LGR Coupler Bracket (Defensemen) (Autodesk Fusion 360 design; units mm, degrees)
Autodesk Fusion 360 part; units mm, degrees
sketch "Sketch1" plane through (0, 0, 0) normal (0, 0, 1) x (1, 0, 0)
  line L0 (-26.575, 21) -> (26.575, 21)
  line L1 (26.575, 21) -> (26.575, -21)
  line L2 (26.575, -21) -> (-26.575, -21)
  line L3 (-26.575, -21) -> (-26.575, 21)
  dimension "d2" = 53.15
  dimension "d3" = 42
  dimension "d4" = 21
  dimension "d5" = 26.575
  constraint horizontal L0
  constraint vertical L1
  constraint horizontal L2
  constraint vertical L3
  measures "d2" distance of L1 L3
  measures "d3" distance of L0 L2
  measures "d4" distance of origin L0
  measures "d5" distance of origin L1
extrude "Extrude1" add sketch "Sketch1" along normal blind 6 makes body 1
sketch "Sketch2" plane through (0, 0, 6) normal (0, 0, 1) x (-1, 0, 0)
  line L0 (26.575, 21) -> (-26.575, 21)
  line L1 (-26.575, 21) -> (-26.575, -21)
  line L2 (-26.575, -21) -> (26.575, -21)
  line L3 (26.575, -21) -> (26.575, 21)
  point P0 (20.01, -13)
  point P1 (-19.99, -13)
  point P2 (20.01, -1)
  point P3 (-19.99, -1)
  dimension "d8" = 40
  dimension "d9" = 12
  dimension "d10" = 6.565
  dimension "d11" = 22
  constraint horizontal P0 P1
  constraint vertical P1 P3
  constraint horizontal P2 P3
  constraint vertical P0 P2
  measures "d8" distance of P0 P1
  measures "d9" distance of P1 P3
  measures "d10" distance of L3 P0
  measures "d11" distance of L0 P2
hole "Hole1" at (-20.01, 13, 6) at (-20.01, 1, 6) at (19.99, 13, 6) at (19.99, 1, 6) direction (0, 0, -1) diameter 5.5 depth 10 tip angle 180 counterbore diameter 10 counterbore depth 5 bodies 1
sketch "Sketch3" plane through (0, 0, 6) normal (0, 0, 1) x (-1, 0, 0)
  circle A0 centre (-19.99, -13) radius 5
  circle A1 centre (20.01, -13) radius 5
  circle A2 centre (20.01, -1) radius 5
  circle A3 centre (-19.99, -1) radius 5
  line L0 (26.575, 21) -> (-26.575, 21)
  line L1 (-26.575, 21) -> (-26.575, -21)
  line L2 (-26.575, -21) -> (26.575, -21)
  line L3 (26.575, -21) -> (26.575, 21)
  circle A4 centre (0.01, -7) radius 12.7
  dimension "d17" = 25.4
  dimension "d18" = 20
  dimension "d19" = 6
  measures "d17" diameter of A4
  measures "d18" horizontal distance of A2.centre A4.centre
  measures "d19" vertical distance of A1.centre A4.centre
extrude "Extrude2" cut sketch "Sketch3" against normal blind 6 contours A4 bodies 1
sketch "Sketch4" plane through (0, 0, 0) normal (0, 0, -1) x (1, 0, 0)
  circle A0 centre (-0.01, -7) radius 12.7
  circle A1 centre (19.99, -13) radius 2.75
  circle A2 centre (-20.01, -13) radius 2.75
  circle A3 centre (-20.01, -1) radius 2.75
  circle A4 centre (19.99, -1) radius 2.75
  line L0 (26.575, 21) -> (-26.575, 21)
  line L1 (-26.575, 21) -> (-26.575, -21)
  line L2 (-26.575, -21) -> (26.575, -21)
  line L3 (26.575, -21) -> (26.575, 21)
  circle A5 centre (-0.01, -7) radius 12.7
  circle A6 centre (-0.01, -7) radius 15.875
  dimension "d22" = 25.4
  dimension "d23" = 31.75
  constraint concentric A0 A5
  constraint concentric A5 A6
  measures "d22" diameter of A5
  measures "d23" diameter of A6
extrude "Extrude3" add sketch "Sketch4" along normal blind 1.25 contours L2 A6 | L2 A6 bodies 1
ref_plane "WorkPlane1" through (0, 0, 49) normal (0, 0, 1) x (1, 0, 0)
sketch "Sketch5" plane through (0, 0, 49) normal (0, 0, 1) x (1, 0, 0)
  line L0 (-28.5, 36) -> (28.5, 36)
  line L1 (28.5, 36) -> (28.5, -21)
  line L2 (28.5, -21) -> (-28.5, -21)
  line L3 (-28.5, -21) -> (-28.5, 36)
  point P0 (-26.575, -21)
  dimension "d27" = 57
  dimension "d28" = 57
  dimension "d29" = 28.5
  constraint horizontal L0
  constraint vertical L1
  constraint horizontal L2
  constraint vertical L3
  constraint horizontal L2.end P0
  measures "d27" distance of L0 L2
  measures "d28" distance of L1 L3
  measures "d29" distance of origin L3
extrude "Extrude4" add sketch "Sketch5" against normal blind 6 separate body makes body 2
sketch "Sketch6" plane through (0, 0, 49) normal (0, 0, 1) x (-1, 0, 0)
  line L0 (28.5, 21) -> (-28.5, 21)
  line L1 (-28.5, 21) -> (-28.5, -36)
  line L2 (-28.5, -36) -> (28.5, -36)
  line L3 (28.5, -36) -> (28.5, 21)
  circle A0 centre (0, -7.5) radius 19.1
  dimension "d32" = 38.2
  dimension "d33" = 28.5
  dimension "d34" = 28.5
  measures "d32" diameter of A0
  measures "d33" distance of L0 A0.centre
  measures "d34" distance of L1 A0.centre
extrude "Extrude5" cut sketch "Sketch6" against normal blind 6 contours A0 bodies 2
sketch "Sketch7" plane through (0, 0, 43) normal (0, 0, -1) x (1, 0, 0)
  circle A0 centre (0, -7.5) radius 19.1
  line L0 (28.5, 21) -> (-28.5, 21)
  line L1 (-28.5, 21) -> (-28.5, -36)
  line L2 (-28.5, -36) -> (28.5, -36)
  line L3 (28.5, -36) -> (28.5, 21)
  line L4 (28.5, -36) -> (18.64, -36)
  line L5 (18.64, -36) -> (18.64, -26.14)
  line L6 (18.64, -26.14) -> (28.5, -26.14)
  line L7 (28.5, -26.14) -> (28.5, -36)
  line L8 (-28.5, -36) -> (-18.64, -36)
  line L9 (-18.64, -36) -> (-18.64, -26.14)
  line L10 (-18.64, -26.14) -> (-28.5, -26.14)
  line L11 (-28.5, -26.14) -> (-28.5, -36)
  line L12 (-28.5, 21) -> (-18.64, 21)
  line L13 (-18.64, 21) -> (-18.64, 11.14)
  line L14 (-18.64, 11.14) -> (-28.5, 11.14)
  line L15 (-28.5, 11.14) -> (-28.5, 21)
  line L16 (28.5, 21) -> (18.64, 21)
  line L17 (18.64, 21) -> (18.64, 11.14)
  line L18 (18.64, 11.14) -> (28.5, 11.14)
  line L19 (28.5, 11.14) -> (28.5, 21)
  dimension "d41" = 9.86
  dimension "d42" = 9.86
  dimension "d43" = 9.86
  dimension "d44" = 9.86
  constraint horizontal L4
  constraint vertical L5
  constraint horizontal L6
  constraint vertical L7
  constraint coincident L2.end L3.start
  constraint horizontal L8
  constraint vertical L9
  constraint horizontal L10
  constraint vertical L11
  constraint coincident L1.end L2.start
  constraint horizontal L12
  constraint vertical L13
  constraint horizontal L14
  constraint vertical L15
  constraint coincident L0.end L1.start
  constraint horizontal L16
  constraint vertical L17
  constraint horizontal L18
  constraint vertical L19
  constraint coincident L0.start L3.end
  constraint horizontal L5.end L9.end
  constraint vertical L5.end L17.end
  constraint horizontal L13.end L17.end
  constraint vertical L9.end L13.end
  measures "d41" distance of L5 L7
  measures "d42" distance of L4 L6
  measures "d43" distance of L16 L18
  measures "d44" distance of L13 L15
sketch "Sketch9" plane through (0, 0, 6) normal (0, 0, 1) x (-1, 0, 0)
  circle A0 centre (0.01, -7) radius 12.7
  circle A1 centre (-19.99, -13) radius 5
  circle A2 centre (20.01, -13) radius 5
  circle A3 centre (20.01, -1) radius 5
  circle A4 centre (-19.99, -1) radius 5
  line L0 (26.575, 21) -> (-26.575, 21)
  line L1 (-26.575, 21) -> (-26.575, -21)
  line L2 (-26.575, -21) -> (26.575, -21)
  line L3 (26.575, -21) -> (26.575, 21)
  line L4 (26.575, -21) -> (21.575, -21)
  line L5 (21.575, -21) -> (21.575, -16)
  line L6 (21.575, -16) -> (26.575, -16)
  line L7 (26.575, -16) -> (26.575, -21)
  line L8 (26.575, 21) -> (21.575, 21)
  line L9 (21.575, 21) -> (21.575, 16)
  line L10 (21.575, 16) -> (26.575, 16)
  line L11 (26.575, 16) -> (26.575, 21)
  line L12 (-26.575, -21) -> (-21.575, -21)
  line L13 (-21.575, -21) -> (-21.575, -16)
  line L14 (-21.575, -16) -> (-26.575, -16)
  line L15 (-26.575, -16) -> (-26.575, -21)
  line L16 (-26.575, 21) -> (-21.575, 21)
  line L17 (-21.575, 21) -> (-21.575, 16)
  line L18 (-21.575, 16) -> (-26.575, 16)
  line L19 (-26.575, 16) -> (-26.575, 21)
  dimension "d45" = 5
  dimension "d46" = 5
  dimension "d47" = 5
  dimension "d48" = 5
  constraint horizontal L4
  constraint vertical L5
  constraint horizontal L6
  constraint vertical L7
  constraint coincident L2.end L3.start
  constraint horizontal L8
  constraint vertical L9
  constraint horizontal L10
  constraint vertical L11
  constraint coincident L0.start L3.end
  constraint horizontal L12
  constraint vertical L13
  constraint horizontal L14
  constraint vertical L15
  constraint coincident L1.end L2.start
  constraint horizontal L16
  constraint vertical L17
  constraint horizontal L18
  constraint vertical L19
  constraint coincident L0.end L1.start
  constraint horizontal L5.end L13.end
  constraint vertical L5.end L9.end
  constraint horizontal L9.end L17.end
  constraint vertical L13.end L17.end
  measures "d45" distance of L5 L7
  measures "d46" distance of L4 L6
  measures "d47" distance of L8 L10
  measures "d48" distance of L17 L19
loft "Loft1" add profiles "Sketch7", "Sketch9" section 1 contours L0 L3 L16 L17 L18 L19 section 2 contours L0 L1 L16 L17 L18 L19 bodies 1 2
loft "Loft2" add profiles "Sketch9", "Sketch7" section 1 contours L0 L3 L8 L9 L10 L11 section 2 contours L0 L1 L12 L13 L14 L15 bodies 1
sketch "Sketch11" plane through (0, 0, 49) normal (0, 0, 1) x (-1, 0, 0)
  circle A0 centre (0, -7.5) radius 19.1
  line L0 (28.5, 21) -> (-28.5, 21)
  line L1 (-28.5, 21) -> (-28.5, -36)
  line L2 (-28.5, -36) -> (28.5, -36)
  line L3 (28.5, -36) -> (28.5, 21)
  point P0 (23.57, -31.07)
  point P1 (-23.57, -31.07)
  point P2 (-23.57, 16.07)
  point P3 (23.57, 16.07)
  dimension "d49" = 47.14
  dimension "d50" = 47.14
  dimension "d51" = 4.93
  dimension "d52" = 4.93
  constraint horizontal P0 P1
  constraint vertical P1 P2
  constraint horizontal P2 P3
  constraint vertical P0 P3
  measures "d49" distance of P0 P1
  measures "d50" distance of P1 P2
  measures "d51" distance of L2 P1
  measures "d52" distance of L1 P1
sketch "Sketch12" plane through (0, 0, 6) normal (0, 0, 1) x (-1, 0, 0)
  line L0 (-26.575, -21) -> (26.575, -21)
  line L1 (26.575, -21) -> (26.575, 16)
  line L2 (26.575, 16) -> (21.575, 16)
  line L3 (21.575, 16) -> (21.575, 21)
  line L4 (21.575, 21) -> (-21.575, 21)
  line L5 (-21.575, 21) -> (-21.575, 16)
  line L6 (-21.575, 16) -> (-26.575, 16)
  line L7 (-26.575, 16) -> (-26.575, -21)
  circle A0 centre (-19.99, -1) radius 5
  circle A1 centre (20.01, -1) radius 5
  circle A2 centre (0.01, -7) radius 12.7
  circle A3 centre (0.01, -7) radius 15.5
  circle A4 centre (20.01, -13) radius 5
  circle A5 centre (-19.99, -13) radius 5
  dimension "d56" = 31
  constraint concentric A2 A3
  measures "d56" diameter of A3
extrude "Extrude6" cut sketch "Sketch12" against normal blind 5 contours L0 A3 | L0 A3 bodies 1
sketch "Sketch13" plane through (0, 0, 49) normal (0, 0, 1) x (-1, 0, 0)
  circle A0 centre (0, -7.5) radius 19.1
  line L0 (28.5, 21) -> (-28.5, 21)
  line L1 (-28.5, 21) -> (-28.5, -36)
  line L2 (-28.5, -36) -> (28.5, -36)
  line L3 (28.5, -36) -> (28.5, 21)
  line L4 (-26.575, 16) -> (-26.575, -21)
  circle A1 centre (19.99, -10.5) radius 5
  circle A2 centre (19.99, 1.5) radius 5
  circle A3 centre (-20.01, -10.5) radius 5
  circle A4 centre (-20.01, 1.5) radius 5
  line L5 (14.99, -10.5) -> (14.99, 1.5)
  line L6 (24.99, -10.5) -> (24.99, 1.5)
  line L7 (-25.01, -10.5) -> (-25.01, 1.5)
  line L8 (-15.01, -10.5) -> (-15.01, 1.5)
  point P0 (-20.01, -10.5)
  point P1 (-20.01, 1.5)
  point P2 (19.99, 1.5)
  point P3 (19.99, -10.5)
  dimension "d59" = 40
  dimension "d60" = 12
  dimension "d62" = 19.5
  dimension "d63" = 6.565
  dimension "d64" = 10
  dimension "d65" = 10
  dimension "d66" = 10
  dimension "d67" = 10
  constraint horizontal P0 P3
  constraint vertical P0 P1
  constraint horizontal P1 P2
  constraint vertical P2 P3
  constraint coincident P3 A1.centre
  constraint coincident P2 A2.centre
  constraint coincident P0 A3.centre
  constraint coincident P1 A4.centre
  constraint coincident A1 L5.start
  constraint coincident A2 L5.end
  constraint tangent A2 L5
  constraint vertical L5
  constraint coincident A1 L6.start
  constraint coincident A2 L6.end
  constraint tangent A2 L6
  constraint parallel L3 L6
  constraint coincident A3 L7.start
  constraint coincident A4 L7.end
  constraint tangent A4 L7
  constraint parallel L6 L7
  constraint coincident A3 L8.start
  constraint coincident A4 L8.end
  constraint tangent A4 L8
  constraint parallel L7 L8
  measures "d59" horizontal distance of P0 P3
  measures "d60" distance of P0 P1
  measures "d62" distance of L0 P1
  measures "d63" distance of P0 L4
  measures "d64" diameter of A1
  measures "d65" diameter of A2
  measures "d66" diameter of A3
  measures "d67" diameter of A4
extrude "Extrude8" cut sketch "Sketch13" against normal blind 6 contours A0 A1 | A0 A1 A2 L6 | A0 A2 | A0 A3 | A0 A3 A4 L7 | A0 A4 picked at (20.3512, -12.1313) picked at (19.7496, 1.4384) picked at (-20.1495, -12.453) picked at (-19.758, 1.4351) bodies 1
extrude "Extrude9" add 1 faces at (13.5638, 21, 4) along direction (0, 1, 0) blind 8.5 on bodies 1 bodies 1
sketch "Sketch14" plane through (0, 0, 6) normal (0, 0, 1) x (-1, 0, 0)
  arc A0 (6.6621, -21) -> (-6.6421, -21) centre (0.01, -7) ccw
  line L0 (6.6621, -21) -> (6.6621, -29.5)
  line L1 (6.6621, -29.5) -> (26.575, -29.5)
  line L2 (26.575, -29.5) -> (26.575, 16)
  line L3 (26.575, 16) -> (21.575, 16)
  line L4 (21.575, 16) -> (21.575, 21)
  line L5 (21.575, 21) -> (-21.575, 21)
  line L6 (-21.575, 21) -> (-21.575, 16)
  line L7 (-21.575, 16) -> (-26.575, 16)
  line L8 (-26.575, 16) -> (-26.575, -29.5)
  line L9 (-26.575, -29.5) -> (-6.6421, -29.5)
  line L10 (-6.6421, -29.5) -> (-6.6421, -21)
  circle A1 centre (-19.99, -1) radius 5
  circle A2 centre (20.01, -1) radius 5
  circle A3 centre (20.01, -13) radius 5
  circle A4 centre (-19.99, -13) radius 5
  circle A5 centre (0.01, -7) radius 15.5
  line L11 (6.6621, -29.5) -> (-6.6421, -29.5)
  line L12 (-6.6421, -21) -> (-6.6421, -29.5)
  line L13 (6.6621, -29.5) -> (6.6621, -21)
  dimension "d74" = 31
  constraint concentric A0 A5
  constraint coincident L0.end L1.start
  constraint coincident L9.end L10.start
  constraint coincident A0.end L10.end
  constraint coincident A0.start L0.start
  measures "d74" diameter of A5
extrude "Extrude10" add sketch "Sketch14" against normal blind 5 contours L0 L10 A5 L11 L12 L13 bodies 1
sketch "Sketch15" plane through (0, 0, 6) normal (0, 0, 1) x (-1, 0, 0)
  line L0 (-26.575, -29.5) -> (26.575, -29.5)
  line L1 (26.575, -29.5) -> (26.575, 16)
  line L2 (26.575, 16) -> (21.575, 16)
  line L3 (21.575, 16) -> (21.575, 21)
  line L4 (21.575, 21) -> (-21.575, 21)
  line L5 (-21.575, 21) -> (-21.575, 16)
  line L6 (-21.575, 16) -> (-26.575, 16)
  line L7 (-26.575, 16) -> (-26.575, -29.5)
  circle A0 centre (0.01, -7) radius 15.5
  circle A1 centre (-19.99, -1) radius 5
  circle A2 centre (20.01, -1) radius 5
  circle A3 centre (20.01, -13) radius 5
  circle A4 centre (-19.99, -13) radius 5
  line L8 (26.575, -29.5) -> (21.575, -29.5)
  line L9 (21.575, -29.5) -> (21.575, -24.5)
  line L10 (21.575, -24.5) -> (26.575, -24.5)
  line L11 (26.575, -24.5) -> (26.575, -29.5)
  line L12 (-26.575, -29.5) -> (-21.575, -29.5)
  line L13 (-21.575, -29.5) -> (-21.575, -24.5)
  line L14 (-21.575, -24.5) -> (-26.575, -24.5)
  line L15 (-26.575, -24.5) -> (-26.575, -29.5)
  dimension "d77" = 5
  dimension "d78" = 5
  dimension "d79" = 5
  constraint horizontal L8
  constraint vertical L9
  constraint horizontal L10
  constraint vertical L11
  constraint coincident L0.end L1.start
  constraint horizontal L12
  constraint vertical L13
  constraint horizontal L14
  constraint vertical L15
  constraint coincident L0.start L7.end
  constraint horizontal L9.end L13.end
  measures "d77" distance of L9 L11
  measures "d78" distance of L8 L10
  measures "d79" distance of L13 L15
loft "Loft5" add profiles "Sketch15", "Sketch7" section 1 contours L0 L7 L12 L13 L14 L15 section 2 contours L2 L3 L4 L5 L6 L7 bodies 1
loft "Loft6" add profiles "Sketch7", "Sketch15" section 1 contours L1 L2 L8 L9 L10 L11 section 2 contours L0 L1 L8 L9 L10 L11 bodies 1
hole "Hole2" at (-23.57, 31.07, 49) at (23.57, 31.07, 49) at (23.57, -16.07, 49) at (-23.57, -16.07, 49) direction (0, 0, -1) diameter 3.85 depth 15 tip angle 180 bodies 1
sketch "Sketch17" plane through (0, 0, 49) normal (0, 0, 1) x (-1, 0, 0)
  circle A0 centre (-23.57, 16.07) radius 1.925
  circle A1 centre (23.57, -31.07) radius 1.925
  circle A2 centre (-23.57, -31.07) radius 1.925
  circle A3 centre (23.57, 16.07) radius 1.925
  arc A4 (17.6095, -14.897) -> (24.99, -10.5) centre (19.99, -10.5) ccw
  arc A5 (-17.6132, -14.8881) -> (17.6095, -14.897) centre (0, -7.5) ccw
  arc A6 (-25.01, -10.5) -> (-17.6132, -14.8881) centre (-20.01, -10.5) ccw
  line L0 (-25.01, -10.5) -> (-25.01, 1.5)
  arc A7 (-15.5006, 3.6599) -> (-25.01, 1.5) centre (-20.01, 1.5) ccw
  arc A8 (15.4886, 3.6765) -> (-15.5006, 3.6599) centre (0, -7.5) ccw
  arc A9 (24.99, 1.5) -> (15.4886, 3.6765) centre (19.99, 1.5) ccw
  line L1 (24.99, 1.5) -> (24.99, -10.5)
  line L2 (28.5, 21) -> (-28.5, 21)
  line L3 (-28.5, 21) -> (-28.5, -36)
  line L4 (-28.5, -36) -> (28.5, -36)
  line L5 (28.5, -36) -> (28.5, 21)
  circle A10 centre (0, -7.5) radius 21
  circle A11 centre (0, -7.5) radius 26
  line L6 (-21.2368, -22.5) -> (0, -7.5)
  line L7 (0, -7.5) -> (21.2368, -22.5)
  arc A12 (-17.1528, -19.6154) -> (-21.2368, -22.5) centre (-19.1948, -21.0577) ccw
  arc A13 (21.2368, -22.5) -> (17.1528, -19.6154) centre (19.1948, -21.0577) ccw
  line L8 (16.6132, 12.5) -> (0, -7.5)
  line L9 (-16.6132, 12.5) -> (0, -7.5)
  arc A14 (13.4184, 8.6538) -> (16.6132, 12.5) centre (15.0158, 10.5769) ccw
  arc A15 (-16.6132, 12.5) -> (-13.4184, 8.6538) centre (-15.0158, 10.5769) ccw
  point P0 (21.2368, -22.5)
  point P1 (-21.2368, -22.5)
  point P2 (17.1528, -19.6154)
  point P3 (-17.1528, -19.6154)
  point P4 (19.1948, -21.0577)
  point P5 (-19.1948, -21.0577)
  point P6 (16.6132, 12.5)
  point P7 (-16.6132, 12.5)
  point P8 (13.4184, 8.6538)
  point P9 (-13.4184, 8.6538)
  point P10 (15.0158, 10.5769)
  point P11 (-15.0158, 10.5769)
  dimension "d87" = 42
  dimension "d88" = 52
  dimension "d89" = 2.5
  dimension "d90" = 15
  dimension "d91" = 20
  dimension "d92" = 2.5
  constraint concentric A5 A10
  constraint concentric A10 A11
  constraint coincident A11 P0
  constraint coincident A11 P1
  constraint horizontal P0 P1
  constraint coincident P1 L6.start
  constraint coincident A5.centre A8.centre
  constraint coincident P0 L7.end
  constraint coincident A10 P2
  constraint coincident L7 P2
  constraint coincident A10 P3
  constraint coincident L6 P3
  constraint coincident L7 P4
  constraint coincident L6 P5
  constraint horizontal P4 P5
  constraint coincident P3 A12.start
  constraint coincident P2 A13.end
  constraint coincident A11 P6
  constraint coincident A11 P7
  constraint coincident P6 L8.start
  constraint coincident P7 L9.start
  constraint coincident L8 P8
  constraint coincident A10 P8
  constraint coincident L9 P9
  constraint coincident A10 P9
  constraint horizontal P6 P7
  constraint coincident L8 P10
  constraint coincident L9 P11
  constraint horizontal P10 P11
  constraint coincident P8 A14.start
  constraint coincident P9 A15.end
  constraint coincident P11 A15.centre
  constraint horizontal P10 A14.centre
  measures "d87" diameter of A10
  measures "d88" diameter of A11
  measures "d89" distance of P3 P5
  measures "d90" vertical distance of A5.centre P1
  measures "d91" vertical distance of A5.centre P7
  measures "d92" distance of P8 P10
extrude "Extrude12" cut sketch "Sketch17" against normal blind 6 contours A10 A11 L6 L7 | L7 A13 | L6 A12 | A10 A11 L8 L9 | L8 A14 | L9 A15 bodies 1
sketch "Sketch18" plane through (0, 0, 6) normal (0, 0, 1) x (-1, 0, 0)
  line L0 (21.575, -24.5) -> (26.575, -24.5)
  line L1 (26.575, -24.5) -> (26.575, 16)
  line L2 (26.575, 16) -> (21.575, 16)
  line L3 (21.575, 16) -> (21.575, 21)
  line L4 (21.575, 21) -> (-21.575, 21)
  line L5 (-21.575, 21) -> (-21.575, 16)
  line L6 (-21.575, 16) -> (-26.575, 16)
  line L7 (-26.575, 16) -> (-26.575, -24.5)
  line L8 (-26.575, -24.5) -> (-21.575, -24.5)
  line L9 (-21.575, -24.5) -> (-21.575, -29.5)
  line L10 (-21.575, -29.5) -> (21.575, -29.5)
  line L11 (21.575, -29.5) -> (21.575, -24.5)
  circle A0 centre (-19.99, -13) radius 5
  circle A1 centre (20.01, -13) radius 5
  circle A2 centre (20.01, -1) radius 5
  circle A3 centre (-19.99, -1) radius 5
  circle A4 centre (0.01, -7) radius 15.5
  line L12 (-2.8725, -27.5) -> (-18.575, -27.5)
  line L13 (-19.575, -26.5) -> (-19.575, -20.9169)
  line L14 (-19.575, -19.5) -> (2.925, -19.5)
  line L15 (2.925, -19.5) -> (2.925, -27.5)
  line L16 (18.575, -27.5) -> (2.8725, -27.5)
  line L17 (-2.925, -27.5) -> (-2.925, -19.5)
  line L18 (-2.925, -19.5) -> (19.575, -19.5)
  line L19 (19.575, -20.9169) -> (19.575, -26.5)
  line L20 (18.24, -19.9747) -> (2.5375, -25.5578)
  line L21 (-2.5375, -25.5578) -> (-18.24, -19.9747)
  arc A5 (18.575, -27.5) -> (19.575, -26.5) centre (18.575, -26.5) ccw
  arc A6 (19.575, -20.9169) -> (18.24, -19.9747) centre (18.575, -20.9169) ccw
  arc A7 (2.5375, -25.5578) -> (2.8725, -27.5) centre (2.8725, -26.5) ccw
  arc A8 (-19.575, -26.5) -> (-18.575, -27.5) centre (-18.575, -26.5) ccw
  arc A9 (-2.8725, -27.5) -> (-2.5375, -25.5578) centre (-2.8725, -26.5) ccw
  arc A10 (-18.24, -19.9747) -> (-19.575, -20.9169) centre (-18.575, -20.9169) ccw
  point P0 (-19.575, -27.5)
  point P1 (19.575, -27.5)
  dimension "d95" = 2
  dimension "d96" = 2
  dimension "d97" = 2
  dimension "d98" = 2
  dimension "d99" = 22.5
  dimension "d100" = 22.5
  dimension "d101" = 8
  dimension "d102" = 8
  dimension "d103" = 1
  dimension "d104" = 1
  constraint horizontal L12
  constraint vertical L13
  constraint horizontal L14
  constraint vertical L15
  constraint horizontal L16
  constraint vertical L17
  constraint horizontal L18
  constraint vertical L19
  constraint coincident P1 L16
  constraint coincident P1 L19
  constraint tangent L16 A5
  constraint tangent L19 A5
  constraint coincident L18.end L20
  constraint coincident L18.end L19
  constraint tangent L20 A6
  constraint tangent L19 A6
  constraint equal A5 A6
  constraint coincident L17.start L20
  constraint coincident L17.start L16
  constraint tangent L20 A7
  constraint tangent L16 A7
  constraint equal A5 A7
  constraint coincident P0 L13
  constraint coincident P0 L12
  constraint tangent L13 A8
  constraint tangent L12 A8
  constraint coincident L15.end L12
  constraint coincident L15.end L21
  constraint tangent L12 A9
  constraint tangent L21 A9
  constraint equal A8 A9
  constraint coincident L14.start L21
  constraint coincident L14.start L13
  constraint tangent L21 A10
  constraint tangent L13 A10
  constraint equal A8 A10
  measures "d95" distance of L11 L19
  measures "d96" distance of L10 L16
  measures "d97" distance of L9 L13
  measures "d98" distance of L10 L12
  measures "d99" distance of P1 L17.start
  measures "d100" distance of L15.end P0
  measures "d101" distance of P1 L18.end
  measures "d102" distance of P0 L14.start
  measures "d103" radius of A5
  measures "d104" radius of A8
extrude "Extrude13" cut sketch "Sketch18" against normal blind 6 contours L12 L17 L21 A9 | L12 L13 L17 L21 A8 A10 | L15 L16 L19 L20 A5 A6 | L15 L16 L20 A7 bodies 1
sketch "Sketch19" plane through (0, 0, 6) normal (0, 0, 1) x (-1, 0, 0)
  line L0 (2.5375, -25.5578) -> (18.24, -19.9747)
  arc A0 (19.575, -20.9169) -> (18.24, -19.9747) centre (18.575, -20.9169) ccw
  line L1 (19.575, -20.9169) -> (19.575, -26.5)
  arc A1 (18.575, -27.5) -> (19.575, -26.5) centre (18.575, -26.5) ccw
  line L2 (18.575, -27.5) -> (2.8725, -27.5)
  arc A2 (2.5375, -25.5578) -> (2.8725, -27.5) centre (2.8725, -26.5) ccw
  line L3 (-18.24, -19.9747) -> (-2.5375, -25.5578)
  arc A3 (-2.8725, -27.5) -> (-2.5375, -25.5578) centre (-2.8725, -26.5) ccw
  line L4 (-2.8725, -27.5) -> (-18.575, -27.5)
  arc A4 (-19.575, -26.5) -> (-18.575, -27.5) centre (-18.575, -26.5) ccw
  line L5 (-19.575, -26.5) -> (-19.575, -20.9169)
  arc A5 (-18.24, -19.9747) -> (-19.575, -20.9169) centre (-18.575, -20.9169) ccw
  line L6 (21.575, -24.5) -> (26.575, -24.5)
  line L7 (26.575, -24.5) -> (26.575, 16)
  line L8 (26.575, 16) -> (21.575, 16)
  line L9 (21.575, 16) -> (21.575, 21)
  line L10 (21.575, 21) -> (-21.575, 21)
  line L11 (-21.575, 21) -> (-21.575, 16)
  line L12 (-21.575, 16) -> (-26.575, 16)
  line L13 (-26.575, 16) -> (-26.575, -24.5)
  line L14 (-26.575, -24.5) -> (-21.575, -24.5)
  line L15 (-21.575, -24.5) -> (-21.575, -29.5)
  line L16 (-21.575, -29.5) -> (21.575, -29.5)
  line L17 (21.575, -29.5) -> (21.575, -24.5)
  circle A6 centre (-19.99, -13) radius 5
  circle A7 centre (20.01, -13) radius 5
  circle A8 centre (20.01, -1) radius 5
  circle A9 centre (-19.99, -1) radius 5
  circle A10 centre (0.01, -7) radius 15.5
  line L18 (19.575, 5) -> (-0.425, 5)
  line L19 (-0.425, 5) -> (-0.425, 19)
  line L20 (2.7474, 19) -> (18.575, 19)
  line L21 (19.575, 18) -> (19.575, 6.9207)
  line L22 (0.425, 5) -> (-19.575, 5)
  line L23 (-19.575, 6.9207) -> (-19.575, 18)
  line L24 (-18.575, 19) -> (-2.7474, 19)
  line L25 (0.425, 19) -> (0.425, 5)
  line L26 (18.0015, 6.1014) -> (2.1739, 17.1808)
  line L27 (-2.1739, 17.1808) -> (-18.0015, 6.1014)
  arc A11 (18.0015, 6.1014) -> (19.575, 6.9207) centre (18.575, 6.9207) ccw
  arc A12 (19.575, 18) -> (18.575, 19) centre (18.575, 18) ccw
  arc A13 (2.7474, 19) -> (2.1739, 17.1808) centre (2.7474, 18) ccw
  arc A14 (-19.575, 6.9207) -> (-18.0015, 6.1014) centre (-18.575, 6.9207) ccw
  arc A15 (-18.575, 19) -> (-19.575, 18) centre (-18.575, 18) ccw
  arc A16 (-2.1739, 17.1808) -> (-2.7474, 19) centre (-2.7474, 18) ccw
  point P0 (19.575, 19)
  point P1 (-19.575, 19)
  dimension "d107" = 2
  dimension "d108" = 2
  dimension "d109" = 2
  dimension "d110" = 14
  dimension "d111" = 14
  dimension "d112" = 20
  dimension "d113" = 20
  dimension "d114" = 1
  dimension "d115" = 1
  constraint horizontal L18
  constraint vertical L19
  constraint horizontal L20
  constraint vertical L21
  constraint horizontal L22
  constraint vertical L23
  constraint horizontal L24
  constraint vertical L25
  constraint horizontal P0 P1
  constraint coincident L18.start L26
  constraint coincident L18.start L21
  constraint tangent L26 A11
  constraint tangent L21 A11
  constraint coincident P0 L20
  constraint coincident P0 L21
  constraint tangent L20 A12
  constraint tangent L21 A12
  constraint equal A11 A12
  constraint coincident L19.end L20
  constraint coincident L19.end L26
  constraint tangent L20 A13
  constraint tangent L26 A13
  constraint equal A11 A13
  constraint coincident L22.end L27
  constraint coincident L22.end L23
  constraint tangent L27 A14
  constraint tangent L23 A14
  constraint coincident P1 L23
  constraint coincident P1 L24
  constraint tangent L23 A15
  constraint tangent L24 A15
  constraint equal A14 A15
  constraint coincident L25.start L24
  constraint coincident L25.start L27
  constraint tangent L24 A16
  constraint tangent L27 A16
  constraint equal A14 A16
  measures "d107" distance of L11 L23
  measures "d108" distance of L10 L24
  measures "d109" distance of L9 L21
  measures "d110" distance of L18.start P0
  measures "d111" distance of L22.end P1
  measures "d112" distance of P1 L25.start
  measures "d113" distance of L19.end P0
  measures "d114" radius of A11
  measures "d115" radius of A14
extrude "Extrude14" cut sketch "Sketch19" against normal blind 6 contours L20 L21 L26 A11 A12 A13 | L23 L24 L27 A14 A15 A16 bodies 1
sketch "Sketch20" plane through (0, 0, 6) normal (0, 0, 1) x (-1, 0, 0)
  line L0 (2.7474, 19) -> (18.575, 19)
  arc A0 (19.575, 18) -> (18.575, 19) centre (18.575, 18) ccw
  line L1 (19.575, 18) -> (19.575, 6.9207)
  arc A1 (18.0015, 6.1014) -> (19.575, 6.9207) centre (18.575, 6.9207) ccw
  line L2 (18.0015, 6.1014) -> (2.1739, 17.1808)
  arc A2 (2.7474, 19) -> (2.1739, 17.1808) centre (2.7474, 18) ccw
  line L3 (-2.1739, 17.1808) -> (-18.0015, 6.1014)
  arc A3 (-19.575, 6.9207) -> (-18.0015, 6.1014) centre (-18.575, 6.9207) ccw
  line L4 (-19.575, 6.9207) -> (-19.575, 18)
  arc A4 (-18.575, 19) -> (-19.575, 18) centre (-18.575, 18) ccw
  line L5 (-18.575, 19) -> (-2.7474, 19)
  arc A5 (-2.1739, 17.1808) -> (-2.7474, 19) centre (-2.7474, 18) ccw
  line L6 (2.5375, -25.5578) -> (18.24, -19.9747)
  arc A6 (19.575, -20.9169) -> (18.24, -19.9747) centre (18.575, -20.9169) ccw
  line L7 (19.575, -20.9169) -> (19.575, -26.5)
  arc A7 (18.575, -27.5) -> (19.575, -26.5) centre (18.575, -26.5) ccw
  line L8 (18.575, -27.5) -> (2.8725, -27.5)
  arc A8 (2.5375, -25.5578) -> (2.8725, -27.5) centre (2.8725, -26.5) ccw
  line L9 (-18.24, -19.9747) -> (-2.5375, -25.5578)
  arc A9 (-2.8725, -27.5) -> (-2.5375, -25.5578) centre (-2.8725, -26.5) ccw
  line L10 (-2.8725, -27.5) -> (-18.575, -27.5)
  arc A10 (-19.575, -26.5) -> (-18.575, -27.5) centre (-18.575, -26.5) ccw
  line L11 (-19.575, -26.5) -> (-19.575, -20.9169)
  arc A11 (-18.24, -19.9747) -> (-19.575, -20.9169) centre (-18.575, -20.9169) ccw
  line L12 (21.575, -24.5) -> (26.575, -24.5)
  line L13 (26.575, -24.5) -> (26.575, 16)
  line L14 (26.575, 16) -> (21.575, 16)
  line L15 (21.575, 16) -> (21.575, 21)
  line L16 (21.575, 21) -> (-21.575, 21)
  line L17 (-21.575, 21) -> (-21.575, 16)
  line L18 (-21.575, 16) -> (-26.575, 16)
  line L19 (-26.575, 16) -> (-26.575, -24.5)
  line L20 (-26.575, -24.5) -> (-21.575, -24.5)
  line L21 (-21.575, -24.5) -> (-21.575, -29.5)
  line L22 (-21.575, -29.5) -> (21.575, -29.5)
  line L23 (21.575, -29.5) -> (21.575, -24.5)
  circle A12 centre (-19.99, -13) radius 5
  circle A13 centre (20.01, -13) radius 5
  circle A14 centre (20.01, -1) radius 5
  circle A15 centre (-19.99, -1) radius 5
  circle A16 centre (0.01, -7) radius 15.5
  line L24 (-18.575, 10.5) -> (-18.575, 19)
  line L25 (-18.575, 19) -> (18.575, 19)
  line L26 (18.575, 19) -> (18.575, 10.5)
  line L27 (14.031, 8.4337) -> (18.0015, 6.1014)
  line L28 (-14.1342, 8.3977) -> (-18.0015, 6.1014)
  line L29 (6.4337, 10.5) -> (-6.4759, 10.5)
  arc A17 (14.031, 8.4337) -> (6.4337, 10.5) centre (6.4337, -4.5) ccw
  arc A18 (-6.4759, 10.5) -> (-14.1342, 8.3977) centre (-6.4759, -4.5) ccw
  dimension "d118" = 2
  dimension "d120" = 15
  dimension "d121" = 15
  constraint vertical L24
  constraint horizontal L25
  constraint vertical L26
  constraint vertical L0.end L26.end
  constraint vertical A4.start L24.start
  constraint coincident A1.start L2.start
  constraint coincident L3.end A3.end
  constraint horizontal L29
  constraint tangent L27 A17
  constraint tangent L29 A17
  constraint tangent L28 A18
  constraint tangent L29 A18
  measures "d118" distance of L16 L25
  measures "d120" radius of A17
  measures "d121" radius of A18
extrude "Extrude15" cut sketch "Sketch20" against normal blind 6 contours L2 A2 L3 A5 L25 L27 L28 L29 A17 A18 bodies 1
sketch "Sketch21" plane through (0, 0, 6) normal (0, 0, 1) x (-1, 0, 0)
  arc A0 (-6.4759, 10.5) -> (-14.1342, 8.3977) centre (-6.4759, -4.5) ccw
  arc A1 (-19.575, 6.9207) -> (-18.0015, 6.1014) centre (-18.575, 6.9207) ccw
  line L0 (-19.575, 6.9207) -> (-19.575, 18)
  arc A2 (-18.575, 19) -> (-19.575, 18) centre (-18.575, 18) ccw
  line L1 (-18.575, 19) -> (18.575, 19)
  arc A3 (19.575, 18) -> (18.575, 19) centre (18.575, 18) ccw
  line L2 (19.575, 18) -> (19.575, 6.9207)
  arc A4 (18.0015, 6.1014) -> (19.575, 6.9207) centre (18.575, 6.9207) ccw
  arc A5 (14.031, 8.4337) -> (6.4337, 10.5) centre (6.4337, -4.5) ccw
  line L3 (6.4337, 10.5) -> (-6.4759, 10.5)
  line L4 (2.5375, -25.5578) -> (18.24, -19.9747)
  arc A6 (19.575, -20.9169) -> (18.24, -19.9747) centre (18.575, -20.9169) ccw
  line L5 (19.575, -20.9169) -> (19.575, -26.5)
  arc A7 (18.575, -27.5) -> (19.575, -26.5) centre (18.575, -26.5) ccw
  line L6 (18.575, -27.5) -> (2.8725, -27.5)
  arc A8 (2.5375, -25.5578) -> (2.8725, -27.5) centre (2.8725, -26.5) ccw
  line L7 (-18.24, -19.9747) -> (-2.5375, -25.5578)
  arc A9 (-2.8725, -27.5) -> (-2.5375, -25.5578) centre (-2.8725, -26.5) ccw
  line L8 (-2.8725, -27.5) -> (-18.575, -27.5)
  arc A10 (-19.575, -26.5) -> (-18.575, -27.5) centre (-18.575, -26.5) ccw
  line L9 (-19.575, -26.5) -> (-19.575, -20.9169)
  arc A11 (-18.24, -19.9747) -> (-19.575, -20.9169) centre (-18.575, -20.9169) ccw
  line L10 (21.575, -24.5) -> (26.575, -24.5)
  line L11 (26.575, -24.5) -> (26.575, 16)
  line L12 (26.575, 16) -> (21.575, 16)
  line L13 (21.575, 16) -> (21.575, 21)
  line L14 (21.575, 21) -> (-21.575, 21)
  line L15 (-21.575, 21) -> (-21.575, 16)
  line L16 (-21.575, 16) -> (-26.575, 16)
  line L17 (-26.575, 16) -> (-26.575, -24.5)
  line L18 (-26.575, -24.5) -> (-21.575, -24.5)
  line L19 (-21.575, -24.5) -> (-21.575, -29.5)
  line L20 (-21.575, -29.5) -> (21.575, -29.5)
  line L21 (21.575, -29.5) -> (21.575, -24.5)
  circle A12 centre (-19.99, -13) radius 5
  circle A13 centre (20.01, -13) radius 5
  circle A14 centre (20.01, -1) radius 5
  circle A15 centre (-19.99, -1) radius 5
  circle A16 centre (0.01, -7) radius 15.5
  circle A17 centre (0.01, -7) radius 17.5
  circle A18 centre (0.01, -7) radius 25
  line L22 (-17.4864, 10.8571) -> (0.01, -7)
  line L23 (0.01, -7) -> (17.5064, 10.8571)
  arc A19 (12.2574, 5.5) -> (17.5064, 10.8571) centre (14.8819, 8.1786) ccw
  arc A20 (-17.4864, 10.8571) -> (-12.2374, 5.5) centre (-14.8619, 8.1786) ccw
  line L24 (18.0015, 6.1014) -> (14.031, 8.4337)
  line L25 (-14.1342, 8.3977) -> (-18.0015, 6.1014)
  point P0 (17.5064, 10.8571)
  point P1 (-17.4864, 10.8571)
  point P2 (12.2574, 5.5)
  point P3 (-12.2374, 5.5)
  point P4 (14.8819, 8.1786)
  point P5 (-14.8619, 8.1786)
  dimension "d124" = 35
  dimension "d125" = 50
  dimension "d126" = 3.75
  dimension "d127" = 12.5
  constraint concentric A16 A17
  constraint concentric A16 A18
  constraint coincident A18 P0
  constraint coincident A18 P1
  constraint horizontal P0 P1
  constraint coincident P1 L22.start
  constraint coincident A16.centre A17.centre
  constraint coincident P0 L23.end
  constraint coincident A17 P2
  constraint coincident L23 P2
  constraint coincident L22 P3
  constraint coincident A17 P3
  constraint coincident L23 P4
  constraint coincident L22 P5
  constraint horizontal P4 P5
  constraint coincident P2 A19.start
  constraint coincident P3 A20.end
  measures "d124" diameter of A17
  measures "d125" diameter of A18
  measures "d126" distance of P0 P4
  measures "d127" vertical distance of A16.centre P2
extrude "Extrude16" cut sketch "Sketch21" against normal blind 6 contours A0 L3 A17 L22 L25 | A5 L3 A17 L23 L24 | L22 A20 L25 | L23 A19 L24 picked at (-16.7906, 6.6089) picked at (16.7998, 6.5967) bodies 1
fillet "Fillet1" radius 100 1 edges at (-18.0033, -6.1002, 3) on bodies 1
fillet "Fillet2" radius 100 1 edges at (17.989, -6.1089, 3) on bodies 1
fillet "Fillet6" radius 2 8 edges at (-23.57, 26.14, 43) (-18.64, 31.07, 43) (-23.57, -11.14, 43) (-18.64, -16.07, 43) (18.64, -16.07, 43) (23.57, -11.14, 43) (23.57, 26.14, 43) (18.64, 31.07, 43) on bodies 1
fillet "Fillet7" radius 2 8 edges at (-21.575, 27, 6) (-24.075, 24.5, 6) (-21.575, -18.5, 6) (-24.075, -16, 6) (21.575, -18.5, 6) (24.075, -16, 6) (24.075, 24.5, 6) (21.575, 27, 6) on bodies 1
fillet "Fillet8" radius 2 20 edges at (-20.9339, -15.2439, 6.7046) (-21.3997, -15.7091, 8.2094) (-20.0909, -13.5425, 24.7093) (-18.7814, -11.3752, 41.2094) (-18.347, -10.9402, 42.2582) (-18.6967, 25.9537, 41.6111) (-18.7959, 26.0491, 41.0349) (-20.1047, 25.3215, 24.5348) (-21.4098, 24.5902, 8.0349) (-20.8511, 24.0277, 6.6131) (20.8511, 24.0277, 6.6131) (21.4098, 24.5902, 8.0349) (20.1047, 25.3215, 24.5348) (18.7959, 26.0491, 41.0349) (18.6967, 25.9537, 41.6111) (18.347, -10.9402, 42.2582) (18.7814, -11.3752, 41.2094) (20.0909, -13.5425, 24.7093) (21.3997, -15.7091, 8.2094) (20.9339, -15.2439, 6.7046) on bodies 1
fillet "Fillet9" radius 2.5 4 edges at (-17.6095, 14.897, 46) (17.6132, 14.8881, 46) (15.5006, -3.6599, 46) (-15.4886, -3.6765, 46) on bodies 1
extrude "Extrude17" add 1 faces at (22.8966, -21, 30.7721) along direction (0, -1, 0) blind 6.5 on bodies 1 bodies 1
sketch "Sketch23" plane through (0, 0, 0) normal (0, 0, -1) x (1, 0, 0)
  arc A0 (18.9983, 6.0147) -> (16.5414, 4.8257) centre (61.3266, -84.5851) ccw
  arc A1 (12.2374, 5.5) -> (16.5414, 4.8257) centre (14.8619, 8.1786) ccw
  arc A2 (12.2374, 5.5) -> (-12.2574, 5.5) centre (-0.01, -7) ccw
  arc A3 (-16.5714, 4.8307) -> (-12.2574, 5.5) centre (-14.8819, 8.1786) ccw
  arc A4 (-16.5714, 4.8307) -> (-19.0012, 6.016) centre (-61.6257, -84.4448) ccw
  arc A5 (-19.575, 6.9207) -> (-19.0012, 6.016) centre (-18.575, 6.9207) ccw
  line L0 (-19.575, 6.9207) -> (-19.575, 18)
  arc A6 (-18.575, 19) -> (-19.575, 18) centre (-18.575, 18) ccw
  line L1 (-18.575, 19) -> (18.575, 19)
  arc A7 (19.575, 18) -> (18.575, 19) centre (18.575, 18) ccw
  line L2 (19.575, 18) -> (19.575, 6.9207)
  arc A8 (18.9983, 6.0147) -> (19.575, 6.9207) centre (18.575, 6.9207) ccw
  circle A9 centre (19.99, -1) radius 2.75
  circle A10 centre (-20.01, -1) radius 2.75
  circle A11 centre (-20.01, -13) radius 2.75
  circle A12 centre (19.99, -13) radius 2.75
  circle A13 centre (-0.01, -7) radius 15.875
  line L3 (26.575, 27.5) -> (-26.575, 27.5)
  line L4 (-26.575, 27.5) -> (-26.575, -29.5)
  line L5 (-26.575, -29.5) -> (26.575, -29.5)
  line L6 (26.575, -29.5) -> (26.575, 27.5)
  line L7 (2.5375, -25.5578) -> (18.24, -19.9747)
  arc A14 (19.575, -20.9169) -> (18.24, -19.9747) centre (18.575, -20.9169) ccw
  line L8 (19.575, -20.9169) -> (19.575, -26.5)
  arc A15 (18.575, -27.5) -> (19.575, -26.5) centre (18.575, -26.5) ccw
  line L9 (18.575, -27.5) -> (2.8725, -27.5)
  arc A16 (2.5375, -25.5578) -> (2.8725, -27.5) centre (2.8725, -26.5) ccw
  line L10 (-18.24, -19.9747) -> (-2.5375, -25.5578)
  arc A17 (-2.8725, -27.5) -> (-2.5375, -25.5578) centre (-2.8725, -26.5) ccw
  line L11 (-2.8725, -27.5) -> (-18.575, -27.5)
  arc A18 (-19.575, -26.5) -> (-18.575, -27.5) centre (-18.575, -26.5) ccw
  line L12 (-19.575, -26.5) -> (-19.575, -20.9169)
  arc A19 (-18.24, -19.9747) -> (-19.575, -20.9169) centre (-18.575, -20.9169) ccw
  line L13 (19.575, 18) -> (-19.575, 18)
  line L14 (-19.575, 18) -> (-19.575, 23.5)
  line L15 (-17.575, 25.5) -> (17.575, 25.5)
  line L16 (19.575, 23.5) -> (19.575, 18)
  arc A20 (19.575, 23.5) -> (17.575, 25.5) centre (17.575, 23.5) ccw
  arc A21 (-17.575, 25.5) -> (-19.575, 23.5) centre (-17.575, 23.5) ccw
  dimension "d160" = 39.15
  dimension "d161" = 2
  dimension "d162" = 2
  constraint horizontal L13
  constraint vertical L14
  constraint horizontal L15
  constraint vertical L16
  constraint coincident A7.start L2.start
  constraint tangent L16 A20
  constraint tangent L15 A20
  constraint tangent L15 A21
  constraint tangent L14 A21
  constraint equal A20 A21
  measures "d160" distance of L14 L16
  measures "d161" distance of L3 L15
  measures "d162" radius of A20
extrude "Extrude18" cut sketch "Sketch23" against normal blind 7 contours A6 L1 A7 L13 | A6 L1 A7 L14 L15 L16 A20 A21 bodies 1
sketch "Sketch24" plane through (0, 0, 49) normal (0, 0, 1) x (-1, 0, 0)
  line L0 (28.5, 27.5) -> (-28.5, 27.5)
  line L1 (-28.5, 27.5) -> (-28.5, -36)
  line L2 (-28.5, -36) -> (28.5, -36)
  line L3 (28.5, -36) -> (28.5, 27.5)
  arc A0 (13.724, 5.7839) -> (17.0102, 5.5151) centre (15.5203, 7.5226) ccw
  arc A1 (24.99, 1.5) -> (17.0102, 5.5151) centre (19.99, 1.5) ccw
  line L4 (24.99, 1.5) -> (24.99, -10.5)
  arc A2 (19.2758, -15.4487) -> (24.99, -10.5) centre (19.99, -10.5) ccw
  arc A3 (19.2758, -15.4487) -> (16.7291, -16.7167) centre (18.9187, -17.9231) ccw
  arc A4 (-16.7304, -16.7143) -> (16.7291, -16.7167) centre (0, -7.5) ccw
  arc A5 (-16.7304, -16.7143) -> (-19.2835, -15.4469) centre (-18.9202, -17.9204) ccw
  arc A6 (-25.01, -10.5) -> (-19.2835, -15.4469) centre (-20.01, -10.5) ccw
  line L5 (-25.01, -10.5) -> (-25.01, 1.5)
  arc A7 (-17.0225, 5.5093) -> (-25.01, 1.5) centre (-20.01, 1.5) ccw
  arc A8 (-17.0225, 5.5093) -> (-13.7314, 5.7762) centre (-15.5287, 7.514) ccw
  arc A9 (13.724, 5.7839) -> (-13.7314, 5.7762) centre (0, -7.5) ccw
  arc A10 (-21.2368, -22.5) -> (21.2368, -22.5) centre (0, -7.5) ccw
  arc A11 (-17.1528, -19.6154) -> (-21.2368, -22.5) centre (-19.1948, -21.0577) ccw
  arc A12 (-17.1528, -19.6154) -> (17.1528, -19.6154) centre (0, -7.5) ccw
  arc A13 (21.2368, -22.5) -> (17.1528, -19.6154) centre (19.1948, -21.0577) ccw
  arc A14 (16.6132, 12.5) -> (-16.6132, 12.5) centre (0, -7.5) ccw
  arc A15 (13.4184, 8.6538) -> (16.6132, 12.5) centre (15.0158, 10.5769) ccw
  arc A16 (13.4184, 8.6538) -> (-13.4184, 8.6538) centre (0, -7.5) ccw
  arc A17 (-16.6132, 12.5) -> (-13.4184, 8.6538) centre (-15.0158, 10.5769) ccw
  circle A18 centre (-23.57, 16.07) radius 1.925
  circle A19 centre (23.57, -31.07) radius 1.925
  circle A20 centre (-23.57, -31.07) radius 1.925
  circle A21 centre (23.57, 16.07) radius 1.925
  line L6 (-17.516, 10) -> (-17.516, 23.5)
  line L7 (-15.516, 25.5) -> (15.516, 25.5)
  line L8 (17.516, 23.5) -> (17.516, 10)
  line L9 (15.0158, 10.5769) -> (-15.0158, 10.5769)
  line L10 (15.0158, 10.5769) -> (17.516, 10.5769)
  line L11 (-15.0158, 10.5769) -> (-17.516, 10.5769)
  arc A22 (17.516, 23.5) -> (15.516, 25.5) centre (15.516, 23.5) ccw
  arc A23 (-15.516, 25.5) -> (-17.516, 23.5) centre (-15.516, 23.5) ccw
  dimension "d165" = 2
  dimension "d166" = 6.054
  dimension "d167" = 6.054
  dimension "d195" = 2
  constraint vertical L6
  constraint horizontal L7
  constraint vertical L8
  constraint coincident A15.centre L9.start
  constraint coincident A17.centre L9.end
  constraint coincident L8 L10.end
  constraint perpendicular L8 L10
  constraint coincident L6 L11.end
  constraint perpendicular L6 L11
  constraint tangent L8 A22
  constraint tangent L7 A22
  constraint tangent L7 A23
  constraint tangent L6 A23
  constraint equal A22 A23
  measures "d165" distance of L0 L7
  measures "d166" distance of A21.centre L8
  measures "d167" distance of A18.centre L6
  measures "d195" radius of A22
extrude "Extrude19" cut sketch "Sketch24" against normal blind 7 contours A14 A15 A17 L6 L7 L8 A22 A23 bodies 1
ref_plane "WorkPlane2" through (28.5, 4.25, 46.026) normal (1, 0, 0) x (0, -1, 0)
sketch "Sketch27" plane through (28.5, 0, 0) normal (1, 0, 0) x (0, 1, 0)
  line L0 (-25.5, 41.5) -> (-25.5, 7)
  line L1 (-24.5, 6) -> (-23.6098, 6)
  line L2 (-22.6166, 6.8837) -> (-18.583, 41.3255)
  line L3 (-20.0728, 43) -> (-24, 43)
  line L4 (36, 49) -> (-27.5, 49)
  line L5 (29.5, 0) -> (-27.5, 0)
  line L6 (-11.3685, 41.2605) -> (-15.7031, 8.2605)
  line L7 (-27.5, 43.052) -> (-27.5, 6.1039)
  arc A0 (-18.583, 41.3255) -> (-20.0728, 43) centre (-20.0728, 41.5) ccw
  arc A1 (-24, 43) -> (-25.5, 41.5) centre (-24, 41.5) ccw
  arc A2 (-25.5, 7) -> (-24.5, 6) centre (-24.5, 7) ccw
  arc A3 (-23.6098, 6) -> (-22.6166, 6.8837) centre (-23.6098, 7) ccw
  point P0 (-22.7201, 6)
  point P1 (-18.3869, 43)
  point P2 (-13.7201, 6)
  point P3 (-9.3855, 43)
  dimension "d179" = 90
  dimension "d180" = 6
  dimension "d181" = 6
  dimension "d184" = 2
  dimension "d186" = 9
  dimension "d189" = 1.5
  dimension "d190" = 1
  constraint vertical L0
  constraint perpendicular L0 L1
  constraint coincident P1 L3
  constraint coincident P1 L2
  constraint tangent L3 A0
  constraint tangent L2 A0
  constraint tangent L0 A1
  constraint tangent L3 A1
  constraint equal A0 A1
  constraint tangent L0 A2
  constraint tangent L1 A2
  constraint coincident P0 L1
  constraint coincident P0 L2
  constraint tangent L1 A3
  constraint tangent L2 A3
  constraint equal A2 A3
  measures "d179" angle of L0 L3
  measures "d180" distance of L3 L4
  measures "d181" distance of L1 L5
  measures "d184" distance of L0 L7
  measures "d186" distance of P0 P2
  measures "d189" radius of A0
  measures "d190" radius of A2
extrude "Extrude21" cut sketch "Sketch27" against normal blind 60 bodies 1
fillet "Fillet15" radius 2 10 edges at (-18.2964, -18.8157, 42.3179) (-18.7777, -18.5928, 41.2421) (-20.095, -20.535, 24.6582) (-21.3446, -22.5453, 7.4926) (-20.3867, -22.9432, 6.2549) (20.3867, -22.9432, 6.2549) (21.3446, -22.5453, 7.4926) (20.095, -20.535, 24.6582) (18.7777, -18.5928, 41.2421) (18.2964, -18.8157, 42.3179) on bodies 1
fillet "Fillet17" radius 2 4 edges at (28.5, 36, 46) (-28.5, 36, 46) (26.575, 29.5, 3) (-26.575, 29.5, 3) on bodies 1
fillet "Fillet18" radius 2 2 edges at (27.2508, 31.7818, 18.9889) (-27.2508, 31.7818, 18.9889) on bodies 1
fillet "Fillet19" radius 1.5 5 edges at (18.149, -25.1446, 42.4695) (18.7649, -25.5, 41.3303) (20.095, -25.5, 24.6582) (21.3609, -25.5, 7.5592) (20.3618, -25.151, 6.2412) on bodies 1
fillet "Fillet19" radius 1.5 5 edges at (-20.3618, -25.151, 6.2412) (-21.3609, -25.5, 7.5592) (-20.095, -25.5, 24.6582) (-18.7649, -25.5, 41.3303) (-18.149, -25.1446, 42.4695) on bodies 1
sketch "Sketch28" plane through (0, 0, 6) normal (0, 0, 1) x (-1, 0, 0)
  line L0 (-19.4101, -27.0501) -> (-19.4101, -29.5)
  line L1 (-19.4101, -29.5) -> (19.4101, -29.5)
  line L2 (19.4101, -29.5) -> (19.4101, -27.0501)
  arc A0 (18.575, -27.5) -> (19.4101, -27.0501) centre (18.575, -26.5) ccw
  line L3 (18.575, -27.5) -> (2.8725, -27.5)
  arc A1 (2.5375, -25.5578) -> (2.8725, -27.5) centre (2.8725, -26.5) ccw
  line L4 (2.5375, -25.5578) -> (18.24, -19.9747)
  arc A2 (19.575, -20.9169) -> (18.24, -19.9747) centre (18.575, -20.9169) ccw
  line L5 (19.575, -20.9169) -> (19.575, -22.5867)
  line L6 (19.575, -22.5867) -> (26.575, -22.5867)
  line L7 (26.575, -22.5867) -> (26.575, 13.7201)
  line L8 (26.575, 13.7201) -> (19.575, 13.7201)
  line L9 (19.575, 13.7201) -> (19.575, 6.9207)
  arc A3 (19.0012, 6.016) -> (19.575, 6.9207) centre (18.575, 6.9207) ccw
  arc A4 (19.0012, 6.016) -> (16.5714, 4.8307) centre (61.6257, -84.4448) ccw
  arc A5 (12.2574, 5.5) -> (16.5714, 4.8307) centre (14.8819, 8.1786) ccw
  arc A6 (12.2574, 5.5) -> (-12.2374, 5.5) centre (0.01, -7) ccw
  arc A7 (-16.5414, 4.8257) -> (-12.2374, 5.5) centre (-14.8619, 8.1786) ccw
  arc A8 (-16.5414, 4.8257) -> (-18.9983, 6.0147) centre (-61.3266, -84.5851) ccw
  arc A9 (-19.575, 6.9207) -> (-18.9983, 6.0147) centre (-18.575, 6.9207) ccw
  line L10 (-19.575, 6.9207) -> (-19.575, 13.7201)
  line L11 (-19.575, 13.7201) -> (-26.575, 13.7201)
  line L12 (-26.575, 13.7201) -> (-26.575, -22.5867)
  line L13 (-26.575, -22.5867) -> (-19.575, -22.5867)
  line L14 (-19.575, -22.5867) -> (-19.575, -20.9169)
  arc A10 (-18.24, -19.9747) -> (-19.575, -20.9169) centre (-18.575, -20.9169) ccw
  line L15 (-18.24, -19.9747) -> (-2.5375, -25.5578)
  arc A11 (-2.8725, -27.5) -> (-2.5375, -25.5578) centre (-2.8725, -26.5) ccw
  line L16 (-2.8725, -27.5) -> (-18.575, -27.5)
  arc A12 (-19.4101, -27.0501) -> (-18.575, -27.5) centre (-18.575, -26.5) ccw
  circle A13 centre (-19.99, -13) radius 5
  circle A14 centre (20.01, -13) radius 5
  circle A15 centre (20.01, -1) radius 5
  circle A16 centre (-19.99, -1) radius 5
  circle A17 centre (0.01, -7) radius 15.5
  circle A18 centre (0.01, -7) radius 17.5
  dimension "d204" = 35
  constraint concentric A6 A18
  measures "d204" diameter of A18
extrude "Extrude22" cut sketch "Sketch28" against normal blind 5 contours A6 A13 A14 A15 A16 A18 bodies 1
fillet "Fillet20" radius 0.5 5 edges at (15.4761, 15.1505, 3.5) (17.4053, 8.7199, 3.5) (17.4053, 5.2801, 3.5) (15.4761, -1.1505, 3.5) (12.2375, -5.5, 3.5) on bodies 1
fillet "Fillet20" radius 0.5 5 edges at (-12.2574, -5.5, 3.5) (-15.4961, -1.1505, 3.5) (-17.4253, 5.2801, 3.5) (-17.4253, 8.7199, 3.5) (-15.4961, 15.1505, 3.5) on bodies 1
extrude "Extrude23" add 1 faces at (23.1953, -22.9983, 49) along direction (0, 0, 1) blind 2 on bodies 1 bodies 1
equation "d4 = ( 42 / 2 ) * 1 mm"
equation "d5 = ( 53.15 / 2 ) * 1 mm"
equation "d10 = ( ( 53.13 - 40 ) / 2 ) * 1 mm"
equation "d26 = 4.9 cm - 6 mm"
equation "d29 = ( 57 / 2 ) * 1 mm"
equation "d33 = ( 57 / 2 ) * 1 mm"
equation "d34 = ( 57 / 2 ) * 1 mm"
equation "d41 = ( 4.93 * 2 ) * 1 mm"
equation "d42 = ( 4.93 * 2 ) * 1 mm"
equation "d43 = ( 4.93 * 2 ) * 1 mm"
equation "d44 = ( 4.93 * 2 ) * 1 mm"
equation "d148 = 1.5 mm + 5 mm"
